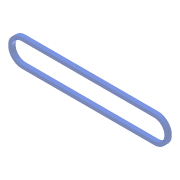
# Autodesk Inventor part: 25 Chain Template
Saved by Autodesk Inventor 2015 (Build 190159000, 159)
## iProperties
Created: 2013-12-27
Part Number: 25 Chain Template
Material: Silicon Nitride
Document SubType Name: Modeling
Designer: Nemo
Density: 3.18 g/cm^3
Appearance: Clear - Blue
Mass: 469.004 g
Surface Area: 851.623 cm^2
Volume: 147.486 cm^3
Author: Nemo
Autodesk Inventor part; units mm, degrees
ref_plane "YZ Plane" through (0, 0, 0) normal (1, 0, 0) x (0, 1, 0)
ref_plane "XZ Plane" through (0, 0, 0) normal (0, 1, 0) x (-1, 0, 0)
ref_plane "XY Plane" through (0, 0, 0) normal (0, 0, 1) x (1, 0, 0)
sketch "Sketch1" plane through (0, 0, 0) normal (0, 0, 1) x (1, 0, 0)
  line L0 (0, 22.2339) -> (247.65, 22.2339) construction
  line L1 (0, -22.2339) -> (247.65, -22.2339) construction
  arc A0 (0, 22.2339) -> (0, -22.2339) centre (0, 0) ccw construction
  line L2 (0, 0) -> (247.65, 0) construction
  arc A1 (247.65, -22.2339) -> (247.65, 22.2339) centre (247.65, 0) ccw construction
  line L3 (247.65, 25.4089) -> (0, 25.4089)
  arc A2 (0, 25.4089) -> (0, -25.4089) centre (0, 0) ccw
  line L4 (0, -25.4089) -> (247.65, -25.4089)
  arc A3 (247.65, -25.4089) -> (247.65, 25.4089) centre (247.65, 0) ccw
  line L5 (247.65, 19.0589) -> (0, 19.0589)
  arc A4 (0, 19.0589) -> (0, -19.0589) centre (0, 0) ccw
  line L6 (0, -19.0589) -> (247.65, -19.0589)
  arc A5 (247.65, -19.0589) -> (247.65, 19.0589) centre (247.65, 0) ccw
  dimension "d1" = 22.234
  dimension "d2" = 22.234
  dimension "d3" = 3.175
  dimension "d4" = 3.175
  dimension "CtoC" = 247.65
  constraints: 14 end point, 12 point on circle, 6 centre point, 4 tangent, 2 coincident, 1 horizontal, 6 other
  measures "d1" radius of A0
  measures "d2" radius of A1
  measures "d3" distance between parallel lines of L3 L0
  measures "d4" distance between parallel lines of L0 L5
  measures "CtoC" distance of L2.start L2.end
extrude "Extrusion1" add sketch "Sketch1" along normal mid plane 7.62
body "Solid1"
